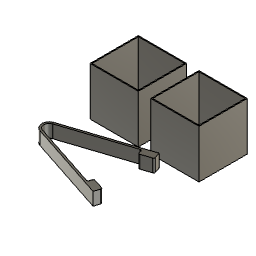
teleop_tong (Autodesk Fusion 360 design; units mm, degrees)
Autodesk Fusion 360 part; units mm, degrees
sketch "Sketch1" plane through (0, 0, 0) normal (0, 0, 1) x (1, 0, 0)
  circle A0 centre (0, 0) radius 10 construction
  line L0 (0, 0) -> (120, 0) construction
  line L1 (120, 0) -> (120, 50) construction
  line L2 (120, 0) -> (120, -50) construction
  line L3 (-3.1247, 9.4993) -> (120, 50) construction
  line L4 (120, -50) -> (-3.1247, -9.4993) construction
  line L5 (-2.656, 8.0744) -> (120.4687, 48.5751)
  line L6 (-3.5934, 10.9242) -> (119.5313, 51.4249)
  circle A1 centre (0, 0) radius 11.5
  circle A2 centre (0, 0) radius 8.5
  line L7 (120.4687, -48.5751) -> (-2.656, -8.0744)
  line L8 (119.5313, -51.4249) -> (-3.5934, -10.9242)
  line L9 (119.5313, -51.4249) -> (120.4687, -48.5751)
  line L10 (119.5313, 51.4249) -> (120.4687, 48.5751)
  line L11 (120.4687, 48.5751) -> (123.1247, 40.5007)
  line L12 (123.1247, 40.5007) -> (104.1261, 34.2513)
  line L13 (104.1261, 34.2513) -> (101.4702, 42.3257)
  line L14 (123.1247, -40.5007) -> (104.1261, -34.2513)
  line L15 (104.1261, -34.2513) -> (101.4702, -42.3257)
  line L16 (120.4687, -48.5751) -> (123.1247, -40.5007)
  dimension "d1" = 20
  dimension "d2" = 120
  dimension "d3" = 50
  dimension "d4" = 50
  dimension "d5" = 1.5
  dimension "d6" = -1.5
  dimension "d7" = 1.5
  dimension "d8" = -1.5
  dimension "d9" = 1.5
  dimension "d10" = -1.5
  dimension "d25" = 8.5
  dimension "d26" = 20
  constraint coincident A0.centre L0.start
  constraint horizontal L0
  constraint perpendicular L0 L1
  constraint perpendicular L0 L2
  constraint coincident A0 L3.start
  constraint coincident A0 L4.end
  constraint tangent A0 L4
  constraint tangent A0 L3
  constraint perpendicular L7 L9
  constraint perpendicular L5 L10
  constraint perpendicular L5 L11
  constraint perpendicular L11 L12
  constraint coincident L5 L13.end
  constraint perpendicular L5 L13
  constraint symmetric L0 L5.end L7.start
  constraint symmetric L0 L11.end L14.start
  constraint symmetric L0 L12.end L14.end
  constraint symmetric L0 L13.end L15.end
  measures "d1" diameter of A0
  measures "d2" distance of A0.centre L0.end
  measures "d3" distance of L0.end L1.end
  measures "d4" distance of L0.end L2.end
  measures "d25" distance of L5.end L11.end
  measures "d26" distance of L11.end L12.end
extrude "Extrude1" add sketch "Sketch1" along normal blind 20 contours L5 L6 A1 L10 | L5 L11 L12 L13 | L5 A1 A2 L7 | A1 L7 L8 L9 | L7 L14 L15 L16 picked at (-2.7316, 10.1109) makes body 1
sketch "Sketch4" plane through (0, 0, 0) normal (0, 0, -1) x (1, 0, 0)
  line L0 (123.1247, 40.5007) -> (119.5313, 51.4249)
  line L1 (119.5313, 51.4249) -> (-3.5934, 10.9242)
  arc A0 (-3.5934, 10.9242) -> (-3.5934, -10.9242) centre (0, 0) ccw
  line L2 (-3.5934, -10.9242) -> (119.5313, -51.4249)
  line L3 (119.5313, -51.4249) -> (123.1247, -40.5007)
  line L4 (123.1247, -40.5007) -> (104.1261, -34.2513)
  line L5 (104.1261, -34.2513) -> (101.4702, -42.3257)
  line L6 (101.4702, -42.3257) -> (-2.656, -8.0744)
  arc A1 (-2.656, 8.0744) -> (-2.656, -8.0744) centre (0, 0) ccw
  line L7 (-2.656, 8.0744) -> (101.4702, 42.3257)
  line L8 (101.4702, 42.3257) -> (104.1261, 34.2513)
  line L9 (104.1261, 34.2513) -> (123.1247, 40.5007)
  line L10 (119.5313, 51.4249) -> (167.0277, 67.0484)
  line L11 (167.0277, 67.0484) -> (143.5924, 138.293)
  line L12 (143.5924, 138.293) -> (72.3479, 114.8577)
  line L13 (72.3479, 114.8577) -> (95.7831, 43.6131)
  line L14 (1.75, 0) -> (22.5, 0)
  line L15 (119.5313, -51.4249) -> (167.0277, -67.0484)
  line L16 (167.0277, -67.0484) -> (143.5924, -138.293)
  line L17 (143.5924, -138.293) -> (72.3479, -114.8577)
  line L18 (72.3479, -114.8577) -> (95.7831, -43.6131)
  dimension "d27" = 50
  dimension "d28" = 75
  dimension "d29" = 75
  constraint coincident L0.end L1.start
  constraint perpendicular L0 L10
  constraint perpendicular L10 L11
  constraint perpendicular L11 L12
  constraint coincident L1 L13.end
  constraint perpendicular L1 L13
  constraint symmetric L0.end L14 L2.end
  constraint symmetric L10.end L14 L15.end
  constraint symmetric L11.end L14 L16.end
  constraint symmetric L12.end L14 L17.end
  constraint symmetric L13.end L14 L18.end
  measures "d27" distance of L0.end L10.end
  measures "d28" distance of L10.end L11.end
  measures "d29" distance of L11.end L12.end
fillet "Fillet4" radius 2 6 edges at (123.1247, -40.5007, 10) (104.1261, -34.2513, 10) (123.1247, 40.5007, 10) (104.1261, 34.2513, 10) (101.4702, -42.3257, 10) (101.4702, 42.3257, 10) on bodies 1
sketch "Sketch5" plane through (0, 0, 0) normal (0, 0, 1) x (1, 0, 0)
  line L0 (0, 63.5819) -> (75, 63.5819)
  line L1 (75, 63.5819) -> (75, 138.5819)
  line L2 (75, 138.5819) -> (0, 138.5819)
  line L3 (0, 138.5819) -> (0, 63.5819)
  line L4 (1.5, 65.0819) -> (73.5, 65.0819)
  line L5 (73.5, 65.0819) -> (73.5, 137.0819)
  line L6 (73.5, 137.0819) -> (1.5, 137.0819)
  line L7 (1.5, 137.0819) -> (1.5, 65.0819)
  dimension "d36" = 75
  dimension "d37" = 75
  dimension "d40" = -1.5
  constraint horizontal L0
  constraint vertical L1
  constraint horizontal L2
  constraint vertical L3
  measures "d36" distance of L0.start L0.end
  measures "d37" distance of L0.start L2.end
extrude "Extrude5" add sketch "Sketch5" along normal blind 1.5 separate body contours L0 L1 L2 L3 | L4 L5 L6 L7 makes body 2
extrude "Extrude6" add sketch "Sketch5" along normal blind 75 separate body makes body 3
combine "Combine1" operation add target body 2 tool bodies 3
copy_body "CopyPasteBodies1" bodies 2 makes body 4
move_body "Move1" bodies 4 to x (1, 0, 0) y (0, 1, 0) z (0, 0, 1) at (94.2711, 0, 0)
